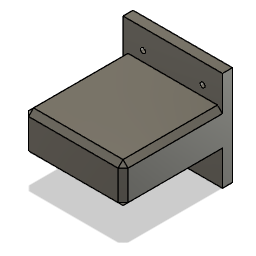
CNC_cable_guide_holder (Autodesk Fusion 360 design; units mm, degrees)
Autodesk Fusion 360 part; units mm, degrees
sketch "Sketch1" plane through (0, 0, 0) normal (0, 0, 1) x (1, 0, 0)
  line L0 (30, 30) -> (-30, 30)
  line L1 (-30, 30) -> (-30, -30)
  line L2 (-30, -30) -> (30, -30)
  line L3 (30, -30) -> (30, 30)
  line L4 (30, 30) -> (-30, -30) construction
  line L5 (-30, 30) -> (30, -30) construction
  circle A0 centre (-30, 30) radius 2.5
  circle A1 centre (30, 30) radius 2.5
  circle A2 centre (-30, -30) radius 2.5
  circle A3 centre (30, -30) radius 2.5
  line L6 (50, 50) -> (-50, 50)
  line L7 (-50, 50) -> (-50, -50)
  line L8 (-50, -50) -> (50, -50)
  line L9 (50, -50) -> (50, 50)
  line L10 (50, 50) -> (-50, -50) construction
  line L11 (-50, 50) -> (50, -50) construction
  line L12 (50, 20) -> (-50, 20)
  line L13 (-50, 20) -> (-50, -20)
  line L14 (-50, -20) -> (50, -20)
  line L15 (50, -20) -> (50, 20)
  line L16 (50, 20) -> (-50, -20) construction
  line L17 (-50, 20) -> (50, -20) construction
  dimension "d1" = 60
  dimension "d2" = 60
  dimension "d3" = 5
  dimension "d6" = 60
  dimension "d7" = -60
  dimension "d8" = 100
  dimension "d9" = 100
  dimension "d10" = 40
  constraint horizontal L0
  constraint perpendicular L0 L1
  constraint parallel L0 L2
  constraint parallel L1 L3
  constraint coincident L4 origin
  constraint coincident L5 origin
  constraint coincident L0.end L1.start
  constraint horizontal L6
  constraint perpendicular L6 L7
  constraint parallel L6 L8
  constraint parallel L7 L9
  constraint coincident L10 origin
  constraint coincident L11 origin
  constraint horizontal L12
  constraint perpendicular L12 L13
  constraint parallel L12 L14
  constraint parallel L13 L15
  constraint coincident L16 origin
  constraint coincident L17 origin
  constraint collinear L9 L15
  measures "d1" distance of L1.end L2.end
  measures "d2" distance of L0.end L1.end
  measures "d3" diameter of A0
  measures "d8" distance of L7.end L8.end
  measures "d9" distance of L6.end L7.end
  measures "d10" distance of L12.end L13.end
extrude "Extrude1" add sketch "Sketch1" along normal blind 10 contours L0 L1 L3 A0 A1 L6 L7 L9 L12 | L0 L1 L3 A0 A1 L12 | L1 L3 L12 L14 | L1 L7 L12 L13 L14 | L3 L9 L12 L14 L15 | L1 L2 L3 A2 A3 L14 | L1 L2 L3 A2 A3 L7 L8 L9 L14
extrude "Extrude2" add sketch "Sketch1" along normal blind 100 from surface at 10 contours L1 L3 L12 L14 | L1 L7 L12 L13 L14 | L3 L9 L12 L14 L15
sketch "Sketch2" plane through (-50, 0, 0) normal (-1, 0, 0) x (0, 0, 1)
  line L0 (0, 50) -> (0, -50)
  line L1 (0, -50) -> (10, -50)
  line L2 (10, -50) -> (10, -20)
  line L3 (10, -20) -> (110, -20)
  line L4 (110, -20) -> (110, 20)
  line L5 (110, 20) -> (10, 20)
  line L6 (10, 20) -> (10, 50)
  line L7 (10, 50) -> (0, 50)
  line L8 (110, -20) -> (10, -20)
  line L9 (10, -20) -> (10, 20)
  line L10 (10, 20) -> (110, 20)
  line L11 (110, 20) -> (110, -20)
  line L12 (23.5, -3) -> (96.5, -3)
  line L13 (102, -3) -> (102, -5)
  line L14 (102, -5) -> (18, -5)
  line L15 (18, -5) -> (18, -3)
  line L16 (60, 20) -> (60, -20)
  line L17 (102, -3) -> (100, -3)
  line L18 (100, 0.5) -> (100, 12)
  line L19 (100, 12) -> (102, 12)
  line L20 (102, 12) -> (102, -3)
  line L21 (20, 0.5) -> (20, 12)
  line L22 (18, 12) -> (18, -3)
  line L23 (20, 12) -> (18, 12)
  line L24 (18, -3) -> (20, -3)
  arc A0 (96.5, -3) -> (100, 0.5) centre (96.5, 0.5) ccw
  arc A1 (20, 0.5) -> (23.5, -3) centre (23.5, 0.5) ccw
  dimension "d16" = 84
  dimension "d17" = 2
  dimension "d18" = 15
  dimension "d19" = 2
  dimension "d20" = 15
  dimension "d21" = 3.5
  constraint horizontal L8
  constraint vertical L9
  constraint horizontal L10
  constraint vertical L11
  constraint coincident L5.end L6.start
  constraint coincident L3.end L4.start
  constraint horizontal L12
  constraint vertical L13
  constraint horizontal L14
  constraint vertical L15
  constraint midpoint L5 L16.start
  constraint midpoint L8 L16.end
  constraint symmetric L13 L15 L16
  constraint horizontal L17
  constraint vertical L18
  constraint horizontal L19
  constraint vertical L20
  constraint symmetric L13.start L16 L15.end
  constraint symmetric L16 L17.end L24.end
  constraint symmetric L16 L18.end L21.end
  constraint symmetric L16 L19.end L22.start
  constraint coincident L13.start L12
  constraint coincident L17.end L18
  constraint tangent L12 A0
  constraint tangent L18 A0
  constraint coincident L15.end L12
  constraint coincident L24.end L21
  constraint tangent L12 A1
  constraint tangent L21 A1
  constraint equal A0 A1
  measures "d16" distance of L15.end L13.start
  measures "d17" distance of L15.end L14.end
  measures "d18" distance of L8 L14
  measures "d19" distance of L13.start L17.end
  measures "d20" distance of L13.start L19.end
  measures "d21" radius of A0
extrude "Extrude3" cut sketch "Sketch2" against normal blind 70 contours L12 L14 L15 L16 L21 L22 L23 A1 | L12 L13 L14 L16 L18 L19 L20 A0
chamfer "Chamfer1" distance 5 angle 45 8 edges at (0, -20, 110) (50, -20, 60) (50, 0, 110) (50, 20, 60) (0, 20, 110) (-50, 20, 60) (-50, 0, 110) (-50, -20, 60)
sketch "Sketch3" plane through (0, 0, 10) normal (0, 0, 1) x (1, 0, 0)
  circle A0 centre (-30, -30) radius 2.5
  circle A1 centre (30, -30) radius 2.5
  line L0 (45, -20) -> (-45, -20)
  line L1 (-45, -20) -> (-50, -15)
  line L2 (-50, -15) -> (-50, -50)
  line L3 (-50, -50) -> (50, -50)
  line L4 (50, -50) -> (50, -15)
  line L5 (50, -15) -> (45, -20)
  line L6 (25, -20) -> (-25, -20)
  line L7 (-25, -20) -> (-25, -50)
  line L8 (-25, -50) -> (25, -50)
  line L9 (25, -50) -> (25, -20)
  dimension "d25" = 50
  dimension "d26" = 25
  constraint horizontal L6
  constraint vertical L7
  constraint horizontal L8
  constraint vertical L9
  constraint coincident L3 L7.end
  constraint coincident L0 L6.start
  measures "d25" distance of L7.end L8.end
  measures "d26" distance of L4 L9
extrude "Extrude4" add sketch "Sketch3" along normal blind 95 contours L0 L3 L6 L7 L8 L9
chamfer "Chamfer2" distance 30 distance2 95 1 edges at (0, -50, 105) measured on face at (-8.3333, -30, 105)
chamfer "Chamfer3" distance 10 distance2 28.6 2 edges at (-25, -35.0055, 57.5017) (25, -35.0055, 57.5017) measured on face at (-8.3333, -40.002, 41.6793) measured on face at (-8.3333, -40.002, 41.6793)
